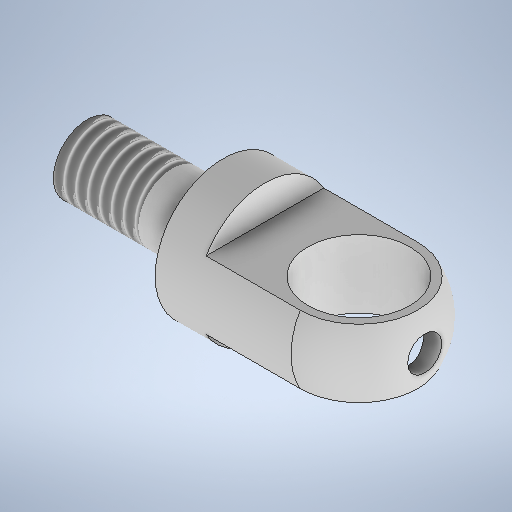
# Autodesk Inventor part: 9
Saved by Autodesk Inventor 2025.1 (Build 291241000, 241)
## iProperties
Created: 2024-09-13
Part Number: 9
Material: Generisch
Document SubType Name: Modeling
Designer: ffogue
Density: 1 g/cm^3
Appearance: Vorgabe
Author: ffogue
Autodesk Inventor part; units mm, degrees
note: some values were not read from the file. Chosen so that the rebuilt part matches the saved one: direction of "Hole1".
ref_plane "XY Plane" through (0, 0, 0) normal (0, 0, 1) x (1, 0, 0)
sketch "Sketch1" plane through (0, 0, 0) normal (0, 0, 1) x (1, 0, 0)
  line L0 (0, 0) -> (0, 2)
  line L1 (0, 2) -> (8, 2)
  line L2 (8, 2) -> (8, 4)
  line L3 (8, 4) -> (16, 4)
  arc A0 (20, 0) -> (16, 4) centre (16, 0) ccw
  line L4 (20, 0) -> (0, 0)
  dimension "d0" = 4
  dimension "d1" = 8
  dimension "d2" = 8
  dimension "d3" = 4
  dimension "d4" = 8
  constraints: 10 end point, 3 perpendicular, 2 point on circle, 1 centre point, 1 parallel, 1 tangent, 1 vertical
  measures "d0" radius of A0
  measures "d1" distance of L0.end L1.end
  measures "d2" distance of L2.end L3.end
  measures "d3" diameter of L1 L4
  measures "d4" diameter of L3 L4
revolve "Revolution1" add sketch "Sketch1" angle 360 about axis through (20, 0, 0) along (-1, 0, 0)
thread "Thread1" size "M4x0.7" class "6g" standard "ISO Metric profile" length 11 offset 3
ref_plane "Work Plane2" through (0, 4, 0) normal (0, 1, 0) x (-1, 0, 0)
sketch "Sketch3" plane through (0, 4, 0) normal (0, 1, 0) x (-1, 0, 0)
  arc A0 (-16, 4) -> (-16, -4) centre (-16, 0) ccw projected
  line L0 (-16, -4) -> (-8, -4) projected
  line L1 (-8, -4) -> (-8, 4) projected
  line L2 (-16, 4) -> (-8, 4) projected
  line L3 (-19.4641, -2) -> (-10.4641, -2)
  line L4 (-10.4641, -2) -> (-10.4641, -4)
  line L5 (-19.4641, 2) -> (-10.4641, 2)
  line L6 (-10.4641, 2) -> (-10.4641, 4)
  point P0 (0, 0)
  dimension "d10" = 9
  dimension "d11" = 4
  dimension "d12" = 2
  constraints: 8 end point, 4 point on line, 2 perpendicular, 2 point on circle, 1 horizontal
  measures "d10" distance of L3.start L3.end
  measures "d11" distance between parallel lines of L5 L3
  measures "d12" distance from line of A0.centre L3
extrude "Extrusion1" cut sketch "Sketch3" against normal blind 8 contours L2 L6 L5 A0 | L3 L4 L0 A0
sketch "Sketch4" plane through (10.4641, -3.4641, 2) normal (0, 0, 1) x (1, 0, 0)
  arc A0 (5.5359, 0) -> (5.5359, 6.9282) centre (5.5359, 3.4641) ccw projected
  point P0 (-10.4641, 3.4641)
  point P1 (5.5359, 3.4641)
  constraints: 1 coincident
hole "Hole1" at (16, 0, 2) direction (0, 0, -1) diameter 6 depth 4
ref_plane "Work Plane3" through (20, 0, 0) normal (1, 0, 0) x (0, 1, 0)
sketch "Sketch5" plane through (20, 0, 0) normal (1, 0, 0) x (0, 1, 0)
  point P0 (0, 0)
  point P1 (0, 0)
  constraints: 1 coincident
hole "Hole2" at (20, 0, 0) direction (-1, 0, 0) diameter 2 depth 2.5
equation "\"d12\" = 0.5 * d11"
body "Solid1"
